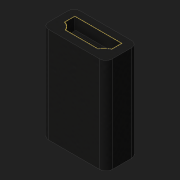
# Autodesk Inventor part: HDMI Port
Saved by Autodesk Inventor 2017 SP1 (Build 210196100, 196)
## iProperties
Created: 2018-03-11
Part Number: HDMI Port
Material: ABS Plastic
Document SubType Name: Modeling
Designer: Zach
Density: 1.06 g/cm^3
Appearance: Black
Author: Zach
Autodesk Inventor part; units mm, degrees
ref_plane "YZ Plane" through (0, 0, 0) normal (1, 0, 0) x (0, 1, 0)
ref_plane "XZ Plane" through (0, 0, 0) normal (0, 1, 0) x (-1, 0, 0)
ref_plane "XY Plane" through (0, 0, 0) normal (0, 0, 1) x (1, 0, 0)
sketch "Sketch1" plane through (0, 0, 0) normal (0, 0, 1) x (1, 0, 0)
  line L0 (0, 0) -> (20, 0)
  line L1 (20, 0) -> (20, 30)
  line L2 (20, 30) -> (0, 30)
  line L3 (0, 30) -> (0, 0)
  dimension "d0" = 20
  dimension "d1" = 30
  constraints: 8 end point, 2 parallel, 1 horizontal, 1 perpendicular
  measures "d0" distance of L2.end L1.end
  measures "d1" distance of L1.end L0.end
extrude "Extrusion1" add sketch "Sketch1" along normal blind 10
fillet "Fillet1" radius 2 4 edges at (0, 15, 10) (20, 15, 10) (20, 15, 0) (0, 15, 0)
sketch "Sketch2" plane through (2, 30, 0) normal (0, 1, 0) x (1, 0, 0)
  line L0 (15.25, -2.5) -> (0.75, -2.5)
  line L1 (0.75, -2.5) -> (0.75, -5.5)
  line L2 (15.25, -2.5) -> (15.25, -5.5)
  line L3 (13, -7.5) -> (3, -7.5)
  line L4 (16, -10) -> (0, -10) projected
  line L5 (8, -2.5) -> (8, -7.5) construction
  line L6 (18, -2) -> (18, -8) projected
  arc A0 (15.25, -5.5) -> (13, -7.5) centre (16.5871, -9.2699) ccw
  arc A1 (3, -7.5) -> (0.75, -5.5) centre (-0.5871, -9.2699) ccw
  point P0 (-2, 0)
  point P1 (8, -10)
  point P2 (8, -5)
  point P3 (18, -5)
  dimension "d5" = 14.5
  dimension "d6" = 3
  dimension "d7" = 2
  dimension "d8" = 10
  dimension "d9" = 4
  dimension "d10" = 4
  constraints: 10 end point, 5 midpoint, 4 point on circle, 2 centre point, 2 horizontal, 2 horizontal alignment, 2 vertical, 2 vertical alignment, 1 perpendicular
  measures "d5" distance of L0.start L0.end
  measures "d6" distance of L0.end L1.end
  measures "d7" vertical distance of L3.end L1.end
  measures "d8" distance of L3.start L3.end
  measures "d9" radius of A0
  measures "d10" radius of A1
extrude "Extrusion2" cut sketch "Sketch2" against normal blind 10
sketch "Sketch3" plane through (2, 20, 0) normal (0, 1, 0) x (1, 0, 0)
  line L0 (0.75, -2.5) -> (15.25, -2.5) projected
  line L1 (0.75, -5.5) -> (0.75, -2.5) projected
  arc A0 (3, -7.5) -> (0.75, -5.5) centre (-0.5871, -9.2699) ccw projected
  line L2 (13, -7.5) -> (3, -7.5) projected
  arc A1 (15.25, -5.5) -> (13, -7.5) centre (16.5871, -9.2699) ccw projected
  line L3 (15.25, -2.5) -> (15.25, -5.5) projected
  arc A2 (2.8734, -7.7) -> (0.55, -5.644) centre (-0.5871, -9.2699) ccw
  line L4 (0.55, -5.644) -> (0.55, -2.3)
  line L5 (0.55, -2.3) -> (15.45, -2.3)
  line L6 (15.45, -2.3) -> (15.45, -5.644)
  arc A3 (15.45, -5.644) -> (13.1266, -7.7) centre (16.5871, -9.2699) ccw
  line L7 (13.1266, -7.7) -> (2.8734, -7.7)
  point P0 (-2, 0)
  dimension "d13" = 0.2
  constraints: 8 end point, 4 point on circle, 2 centre point, 5 other
  measures "d13" distance between parallel lines of L2 L7
extrude "Extrusion3" add sketch "Sketch3" along normal blind 10.1
sketch "Sketch4" plane through (2, 20, 0) normal (0, 1, 0) x (1, 0, 0)
  line L0 (13.5, -5) -> (2.5, -5)
  line L1 (2.5, -5) -> (2.5, -4)
  line L2 (2.5, -4) -> (13.5, -4)
  line L3 (13.5, -4) -> (13.5, -5)
  line L4 (13, -7.5) -> (3, -7.5) projected
  line L5 (0.75, -2.5) -> (15.25, -2.5) projected
  point P0 (-2, 0)
  point P1 (8, -5)
  point P2 (8, -7.5)
  dimension "d16" = 11
  dimension "d17" = 1
  dimension "d18" = 1.5
  constraints: 8 end point, 2 midpoint, 2 parallel, 1 horizontal, 1 perpendicular, 1 vertical alignment
  measures "d16" distance of L1.end L2.end
  measures "d17" distance of L0.end L1.end
  measures "d18" distance between parallel lines of L5 L2
extrude "Extrusion4" add sketch "Sketch4" along normal blind 8
body "Solid1"
